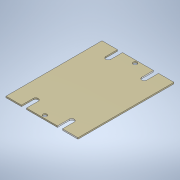
# Autodesk Inventor part: etl standard baseplate with cutouts
Saved by Autodesk Inventor 2022 (Build 260153000, 153)
## iProperties
Created: 2021-07-27
Part Number: etl standard baseplate with cutouts
Material: Generic
Document SubType Name: Modeling
Designer: Caleb
Density: 1 g/cm^3
Appearance: Default
Sending System: Autodesk Inventor 2022
Preprocessor: ST-DEVELOPER v18.1
Title: C:\Users\Caleb\Desktop\etl standard baseplate.stp
Author: Caleb
Autodesk Inventor part; units mm, degrees
ref_plane "YZ Plane" through (0, 0, 0) normal (1, 0, 0) x (0, 1, 0)
ref_plane "XZ Plane" through (0, 0, 0) normal (0, 1, 0) x (-1, 0, 0)
ref_plane "XY Plane" through (0, 0, 0) normal (0, 0, 1) x (1, 0, 0)
sketch "Sketch2" plane through (0, 0, 0) normal (0, 1, 0) x (-1, 0, 0)
  line L0 (-21.55, -28.75) -> (21.55, -28.75)
  line L1 (21.55, -28.75) -> (21.55, 28.75)
  line L2 (21.55, 28.75) -> (-21.55, 28.75)
  line L3 (-21.55, 28.75) -> (-21.55, -28.75)
  line L4 (-21.55, -28.75) -> (21.55, 28.75) construction
  line L5 (21.55, -28.75) -> (-21.55, 28.75) construction
  point P0 (0, 0)
  dimension "d28" = 43.1
  dimension "d29" = 57.5
  constraints: 12 end point, 2 midpoint, 2 parallel, 1 horizontal, 1 perpendicular
  measures "d28" distance of L1.end L2.end
  measures "d29" distance of L0.end L1.end
extrude "Extrusion2" add sketch "Sketch2" along normal blind 0.8
sketch "Sketch3" plane through (0, 0.8, 0) normal (0, 1, 0) x (1, 0, 0)
  line L0 (21.55, 28.75) -> (-21.55, 28.75) projected
  line L1 (3.17, 0) -> (-3.4256, 0) construction
  line L2 (-12.275, -28.75) -> (-12.275, -21.75)
  line L3 (-9.275, -21.75) -> (-9.275, -28.75)
  arc A0 (-9.275, -21.75) -> (-12.275, -21.75) centre (-10.775, -21.75) ccw
  line L4 (-21.55, -28.75) -> (21.55, -28.75) projected
  line L5 (-12.275, 28.75) -> (-12.275, 21.75)
  line L6 (-9.275, 21.75) -> (-9.275, 28.75)
  arc A1 (-12.275, 21.75) -> (-9.275, 21.75) centre (-10.775, 21.75) ccw
  line L7 (-21.55, 28.75) -> (21.55, 28.75)
  line L8 (-21.55, 28.75) -> (-21.55, -28.75) projected
  line L9 (0, -17.1625) -> (0, 19.373) construction
  line L10 (12.275, -28.75) -> (12.275, -21.75)
  line L11 (9.275, -21.75) -> (9.275, -28.75)
  arc A2 (12.275, -21.75) -> (9.275, -21.75) centre (10.775, -21.75) ccw
  line L12 (12.275, 28.75) -> (12.275, 21.75)
  line L13 (9.275, 21.75) -> (9.275, 28.75)
  arc A3 (9.275, 21.75) -> (12.275, 21.75) centre (10.775, 21.75) ccw
  line L14 (21.55, 28.75) -> (-21.55, 28.75)
  point P0 (0, 0)
  dimension "d32" = 3
  dimension "d33" = 7
  dimension "d34" = 1.5
  dimension "d48" = 10.775
  constraints: 24 end point, 17 symmetric about line, 8 point on circle, 6 point on line, 4 centre point, 2 parallel, 1 horizontal, 1 perpendicular, 1 vertical, 3 other
  measures "d32" distance between parallel lines of L2 L3
  measures "d33" distance of L2.start L2.end
  measures "d34" radius of A0
  measures "d48" distance from line of L8 A0.centre
extrude "Extrusion3" cut sketch "Sketch3" against normal through all
sketch "Sketch4" plane through (0, 0.8, 0) normal (0, 1, 0) x (1, 0, 0)
  line L0 (-21.55, 28.75) -> (-21.55, -28.75) projected
  line L1 (-21.55, -28.75) -> (21.55, -28.75) projected
  line L2 (21.55, -28.75) -> (21.55, 28.75) projected
  line L3 (21.55, 28.75) -> (-21.55, 28.75) projected
  point P0 (0, 0)
  point P1 (0, -27)
  point P2 (0, 27)
  point P3 (-12.275, -28.75)
  point P4 (-12.275, 28.75)
  dimension "d37" = 21.55
  dimension "d38" = 1.75
  dimension "d40" = 1.75
  constraints: 1 vertical alignment
  measures "d37" distance from line of L0 point (0, -27)
  measures "d38" distance from line of L1 point (0, -27)
  measures "d40" distance from line of L3 point (0, 27)
hole "Hole1" at (0, 0.8, 27) at (0, 0.8, -27) direction (0, -1, 0) diameter 2.4 end through all clearance for "Flat Head Machine Screw" size "M2" standard "Ansi Metric M Profile"
equation "\"d40\" = d38"
body "Solid3"
